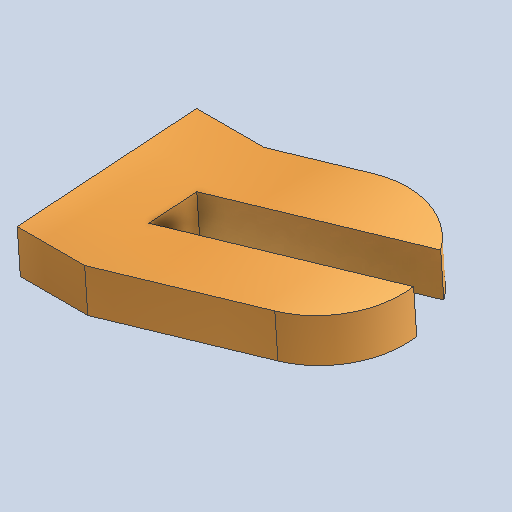
# Autodesk Inventor part: aux_nose_bottom_bracket
Saved by Autodesk Inventor 2022 (Build 260153070, 153G)
## iProperties
Created: 2021-04-29
Part Number: aux_nose_bottom_bracket
Material: Plywood, Sheathing, Glazed
Document SubType Name: Modeling
Designer: kardo
Density: 0.75 g/cm^3
Appearance: Plywood - New(2)
Mass: 0.100239 g
Surface Area: 2.4115 cm^2
Volume: 0.133652 cm^3
Author: kardo
Autodesk Inventor part; units mm, degrees
ref_plane "YZ Plane" through (0, 0, 0) normal (1, 0, 0) x (0, 1, 0)
ref_plane "XZ Plane" through (0, 0, 0) normal (0, 1, 0) x (-1, 0, 0)
ref_plane "XY Plane" through (0, 0, 0) normal (0, 0, 1) x (1, 0, 0)
derived "frame_outline.ipt"
sketch "joints" plane through (81, 0, 0) normal (1, 0, 0) x (0, 1, 0)
  line L0 (-37.9005, 25.6108) -> (-277.6703, 19.7906) construction
  line L1 (94.8, 28.832) -> (28.4595, 27.2216) construction
  line L2 (28.4595, 27.2216) -> (-37.9005, 25.6108) construction
  line L3 (-363, 18.496) -> (-297.6664, 19.4083) construction
  line L4 (-121, 716.7765) -> (-121, -158.9765) construction
  line L5 (-242, 716.7765) -> (-242, -158.9765) construction
  line L6 (237, 716.7765) -> (237, -158.9765) construction
  line L7 (-363, 716.7765) -> (-363, -158.9765) construction
  line L8 (143.2909, -175.9483) -> (77.9563, 758.3799) construction
  line L9 (0, 0) -> (130.35, 9.115) construction
  line L10 (0, 716.7765) -> (0, -158.9765) construction
  line L11 (-242, 46.7048) -> (-242, 33.6806) construction
  line L12 (-242, 33.6806) -> (-242, 20.6564) construction
  line L13 (-363, 38.08) -> (-363, 28.288) construction
  line L14 (-363, 28.288) -> (-363, 18.496) construction
  line L15 (-121, 51.5188) -> (-121, 37.5562) construction
  line L16 (-121, 37.5562) -> (-121, 23.5936) construction
  line L17 (0, 54.4) -> (0, 40.4654) construction
  line L18 (0, 40.4654) -> (0, 26.5308) construction
  line L19 (94.8, 37.536) -> (94.8, 33.184) construction
  line L20 (94.8, 33.184) -> (94.8, 28.832) construction
  line L21 (94.8, 37.536) -> (94.8, 28.832) construction
  line L22 (130.35, 9.115) -> (129.7793, 17.2757) construction
  line L23 (129.7793, 17.2757) -> (129.2087, 25.4364) construction
  line L24 (129.2087, 25.4364) -> (128.638, 33.5972) construction
  line L25 (128.638, 33.5972) -> (128.0674, 41.7579) construction
  line L26 (128.0674, 41.7579) -> (127.4967, 49.9186) construction
  spline S0 degree 3 poles (-363, 38.08) (-277.2033, 46.9603) (-131.9759, 52.0964) (0, 54.4) knots 0 0 0 0 1 1 1 1 construction
  spline S1 degree 3 poles (-297.6664, 19.4083) (-291.0004, 19.5014) (-284.3349, 19.6288) (-277.6703, 19.7906) knots 0 0 0 0 1 1 1 1 construction
  spline S2 degree 4 poles (0, 54.4) (23.3745, 54.808) (84.9613, 55.883) (149.0088, 47.5461) (201.9993, 42.6196) (237, 36.448) knots 0 0 0 0 0 0.379537 1 1 1 1 1 construction
  spline S3 degree 3 poles (130.35, 9.115) (172.0992, 12.0344) (220.2053, 21.9532) (237, 36.448) knots 0 0 0 0 1 1 1 1 construction
sketch "joints_nose" plane through (84, 0, 0) normal (1, 0, 0) x (0, 1, 0)
  line L0 (129.046, 27.7634) -> (235.7442, 35.2245) construction
  line L1 (128.6952, 32.7794) -> (236.1697, 36.5325) construction
  line L2 (195.9322, 35.1273) -> (196.0258, 32.4471) construction
  line L3 (196.2351, 29.4544) -> (196.0258, 32.4471)
  line L4 (196.0258, 32.4471) -> (195.8863, 34.4422)
  line L5 (195.8863, 34.4422) -> (195.677, 37.4349)
  line L6 (203.8226, 38.4047) -> (203.9273, 35.4065)
  line L7 (203.9971, 33.4077) -> (204.1018, 30.4096)
  line L8 (203.9273, 35.4065) -> (203.9971, 33.4077)
  point P0 (0, 0)
ref_plane "plane_stringer_outer" through (84, 0, 0) normal (1, 0, 0) x (0, 1, 0)
ref_plane "plane_sponson_edge_bottom" through (81, 0, 19.8753) normal (-0.3533007, 0.0652579, -0.933231) x (0.9352244, 0, -0.3540554)
sketch "Sketch3" plane through (84, 0, 0) normal (1, 0, 0) x (0, 1, 0)
  line L0 (128.6952, 32.7794) -> (236.1697, 36.5325) construction
  line L1 (129.046, 27.7634) -> (235.7442, 35.2245) construction
  line L2 (195.677, 37.4349) -> (196.2351, 29.4544)
  line L3 (196.2351, 29.4544) -> (194.2399, 29.3149)
  line L4 (194.2399, 29.3149) -> (193.6819, 37.2954)
  line L5 (193.6819, 37.2954) -> (195.677, 37.4349)
  point P0 (0, 0)
  point P1 (203.9273, 35.4065)
  point P2 (196.0258, 32.4471)
  dimension "d12" = 2
  constraints: 8 end point, 2 parallel, 1 perpendicular
  measures "d12" distance of L4.end L2.start
extrude "Extrusion2" add sketch "Sketch3" against normal blind 3
sketch "Sketch6" plane through (81, 196.2351, 29.4544) normal (0, 0.9975641, 0.0697565) x (1, 0, 0)
  line L0 (-115.8411, -47.881) -> (46.3137, 13.3577) projected
  line L1 (3, 0) -> (3, -8) projected
  line L2 (3, 0) -> (0, 0) projected
  line L3 (0, -8) -> (0, 0) projected
  line L4 (3, -8) -> (0, -8) projected
  line L5 (3, -8) -> (3, 0) projected
  line L6 (3, -8) -> (12.6456, -4.3573)
  line L7 (12.6456, -4.3573) -> (10.0014, 2.6441)
  line L8 (10.0014, 2.6441) -> (3, 0)
  point P0 (-81, 15.694)
  constraints: 6 end point, 2 parallel, 2 perpendicular
extrude "Extrusion4" add sketch "Sketch6" against normal up to surface (2 mm away) contours L1 L8 L7 L0 | L0 L7 L6 L1
full round fillet "Full Round Fillet1" first side at (87.2152, 195.0967, 36.1771) centre faces at (92.7642, 195.4289, 31.4264) second side at (88.6676, 195.693, 27.6494)
sketch "Sketch8" plane through (81, 196.2351, 29.4544) normal (0, 0.9975641, 0.0697565) x (1, 0, 0)
  line L0 (-115.8411, -47.881) -> (46.3137, 13.3577) projected
  line L1 (3, -3) -> (3, -5.1379)
  line L2 (3, -5.1379) -> (11.5549, -1.907)
  arc A0 (9.1448, -5.6794) -> (6.5007, 1.3221) centre (7.8228, -2.1786) ccw projected
  point P0 (-81, 15.694)
  point P1 (3, -8)
  point P2 (3, 0)
  point P3 (10.8818, -0.0234)
  dimension "d15" = 2
  constraints: 4 end point, 3 point on line, 1 parallel, 1 point on circle
  measures "d15" distance between parallel lines of L2 L0
extrude "Extrusion5" cut sketch "Sketch8" along normal through all both and the other way through all
equation "\"d12\" = bulkhead_thickness"
equation "\"d7\" = stringer_thickness"
equation "\"d13\" = stringer_thickness"
equation "\"d15\" = bulkhead_thickness"
equation "\"bulkhead_thickness\" = 2"
equation "\"stringer_thickness\" = 3"
body "Solid1"
